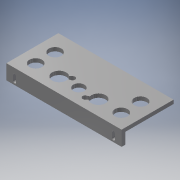
# Autodesk Inventor part: frontPanel
Saved by Autodesk Inventor 2017 (Build 210142000, 142)
## iProperties
Created: 2019-11-20
Part Number: frontPanel
Material: S235
Document SubType Name: Modeling
Designer: Casper
Density: 7.86 g/cm^3
Appearance: Steel
Author: Casper
Autodesk Inventor part; units mm, degrees
ref_plane "YZ Plane" through (0, 0, 0) normal (1, 0, 0) x (0, 1, 0)
ref_plane "XZ Plane" through (0, 0, 0) normal (0, 1, 0) x (-1, 0, 0)
ref_plane "XY Plane" through (0, 0, 0) normal (0, 0, 1) x (1, 0, 0)
sketch "Sketch1" plane through (0, 0, 0) normal (0, 0, 1) x (1, 0, 0)
  line L0 (-77.5, -35) -> (77.5, -35)
  line L1 (77.5, -35) -> (77.5, 35)
  line L2 (77.5, 35) -> (-77.5, 35)
  line L3 (-77.5, 35) -> (-77.5, -35)
  line L4 (-77.5, -35) -> (77.5, 35) construction
  line L5 (77.5, -35) -> (-77.5, 35) construction
  point P0 (0, 0)
  dimension "d23" = 155
  dimension "d24" = 70
  constraints: 12 end point, 2 midpoint, 2 parallel, 1 horizontal, 1 perpendicular
  measures "d23" distance of L0.start L0.end
  measures "d24" distance of L2.end L0.start
extrude "Extrusion2" add sketch "Sketch1" along normal blind 5
sketch "Sketch2" plane through (0, 0, 5) normal (0, 0, 1) x (1, 0, 0)
  line L0 (-77.5, -35) -> (77.5, -35) projected
  line L1 (77.5, -35) -> (77.5, 35) projected
  line L2 (77.5, 35) -> (-77.5, 35) projected
  line L3 (-77.5, 35) -> (-77.5, -35) projected
  line L4 (-77.5, -15) -> (77.5, -15) construction
  line L5 (77.5, -35) -> (77.5, 35) construction
  circle A0 centre (0, -15) radius 7.5
  circle A1 centre (26.5, -15) radius 9.5
  line L6 (0, 35) -> (0, -35) construction
  line L7 (-77.5, -35) -> (77.5, -35) construction
  circle A2 centre (-26.5, -15) radius 9.5
  circle A3 centre (15.5455, -22) radius 3.5
  circle A4 centre (-15.5455, -8) radius 3.5
  point P0 (0, 0)
  dimension "d27" = 20
  dimension "d28" = 15
  dimension "d29" = 19
  dimension "d30" = 26.5
  dimension "d31" = 7
  dimension "d32" = 7
  dimension "d33" = 7
  constraints: 5 centre point, 4 end point, 3 midpoint, 3 point on line, 2 tangent, 1 equal radius, 1 perpendicular, 1 symmetric about line, 1 other
  measures "d27" distance between parallel lines of L0 L4
  measures "d28" diameter of A0
  measures "d29" diameter of A1
  measures "d30" distance of A1.centre A0.centre
  measures "d31" diameter of A4
  measures "d32" vertical distance of A4.centre A2.centre
  measures "d33" vertical distance of A1.centre A3.centre
extrude "Extrusion3" cut sketch "Sketch2" against normal through all contours A0 | A1 | A3 | A2 | A4
sketch "Sketch3" plane through (0, 0, 5) normal (0, 0, 1) x (1, 0, 0)
  circle A0 centre (-26.5, -15) radius 9.5 projected
  circle A1 centre (-15.5455, -8) radius 3.5 projected
  circle A2 centre (26.5, -15) radius 9.5 projected
  circle A3 centre (15.5455, -22) radius 3.5 projected
  circle A4 centre (0, -15) radius 7.5 projected
  line L0 (-77.5, -35) -> (77.5, -35) projected
  line L1 (77.5, -35) -> (77.5, 35) projected
  line L2 (77.5, 35) -> (-77.5, 35) projected
  line L3 (-77.5, 35) -> (-77.5, -35) projected
  circle A5 centre (-26.5, -15) radius 9.5 projected
  line L4 (-20.5198, -7.6184) -> (-18.68, -6.4428)
  circle A6 centre (-15.5455, -8) radius 3.5 projected
  line L5 (-15.5455, -8) -> (-26.5, -15) construction
  line L6 (15.5455, -22) -> (26.5, -15) construction
  circle A7 centre (15.5455, -22) radius 3.5 projected
  line L7 (15.4493, -18.5013) -> (17.2891, -17.3257)
  line L8 (-17.2891, -12.6743) -> (-15.4493, -11.4987)
  line L9 (18.68, -23.5572) -> (20.5198, -22.3816)
  point P0 (0, 0)
  point P1 (-18.4948, -9.8846)
  point P2 (18.4948, -20.1154)
  dimension "d36" = 3
  dimension "d37" = 3
  dimension "d38" = 3
  dimension "d39" = 3
  constraints: 14 point on circle, 12 end point, 4 parallel
  measures "d36" distance between parallel lines of L4 L5
  measures "d37" distance between parallel lines of L7 L6
  measures "d38" distance between parallel lines of L8 L5
  measures "d39" distance between parallel lines of L9 L6
extrude "Extrusion4" cut sketch "Sketch3" against normal through all contours A0 A1 L8 | L4 A1 A0 | A2 A3 L7 | L9 A3 A2
sketch "Sketch4" plane through (0, 0, 5) normal (0, 0, 1) x (1, 0, 0)
  line L0 (-15.4493, -11.4987) -> (-17.2891, -12.6743) projected
  arc A0 (-20.5198, -7.6184) -> (-17.2891, -12.6743) centre (-26.5, -15) ccw projected
  line L1 (-20.5198, -7.6184) -> (-18.68, -6.4428) projected
  arc A1 (-15.4493, -11.4987) -> (-18.68, -6.4428) centre (-15.5455, -8) ccw projected
  line L2 (15.4493, -18.5013) -> (17.2891, -17.3257) projected
  arc A2 (20.5198, -22.3816) -> (17.2891, -17.3257) centre (26.5, -15) ccw projected
  line L3 (20.5198, -22.3816) -> (18.68, -23.5572) projected
  arc A3 (15.4493, -18.5013) -> (18.68, -23.5572) centre (15.5455, -22) ccw projected
  circle A4 centre (0, -15) radius 7.5 projected
  line L4 (-77.5, -35) -> (77.5, -35) projected
  line L5 (77.5, -35) -> (77.5, 35) projected
  line L6 (77.5, 35) -> (-77.5, 35) projected
  line L7 (-77.5, 35) -> (-77.5, -35) projected
  line L8 (-77.5, -25) -> (77.5, -25) construction
  line L9 (-67.5, -25) -> (-47.5, -25) construction
  line L10 (-47.5, -25) -> (-47.5, 20) construction
  line L11 (-47.5, 20) -> (-67.5, 20) construction
  line L12 (-67.5, 20) -> (-67.5, -25) construction
  line L13 (77.5, 35) -> (-77.5, 35) construction
  line L14 (0, 35) -> (0, -35) construction
  circle A5 centre (-57.5, 10.5) radius 8.5
  circle A6 centre (-57.5, -15.5) radius 8.5
  line L15 (-67.5, -2.5) -> (-47.5, -2.5) construction
  line L16 (-57.5, -2.5) -> (-57.5, 10.5) construction
  line L17 (-57.5, -2.5) -> (-57.5, -15.5) construction
  circle A7 centre (57.5, 10.5) radius 8.5
  circle A8 centre (57.5, -15.5) radius 8.5
  point P0 (0, 0)
  dimension "d42" = 10
  dimension "d43" = 10
  dimension "d44" = 20
  dimension "d45" = 45
  dimension "d46" = 17
  dimension "d48" = 26
  constraints: 18 end point, 5 midpoint, 4 centre point, 3 point on line, 2 parallel, 2 perpendicular, 2 symmetric about line, 2 vertical, 1 collinear, 1 equal radius, 1 horizontal, 2 other
  measures "d42" distance between parallel lines of L4 L8
  measures "d43" distance between parallel lines of L7 L12
  measures "d44" distance of L10.end L11.end
  measures "d45" distance of L9.end L10.end
  measures "d46" diameter of A5
  measures "d48" distance of L17.end L16.end
extrude "Extrusion5" cut sketch "Sketch4" against normal through all contours A5 | A6 | A7 | A8
sketch "Sketch5" plane through (0, 0, 0) normal (0, 0, -1) x (-1, 0, 0)
  circle A0 centre (-57.5, 10.5) radius 8.5 projected
  circle A1 centre (57.5, 10.5) radius 8.5 projected
  circle A2 centre (57.5, -15.5) radius 8.5 projected
  circle A3 centre (-57.5, -15.5) radius 8.5 projected
  line L0 (17.2891, -12.6743) -> (15.4493, -11.4987) projected
  arc A4 (18.68, -6.4428) -> (15.4493, -11.4987) centre (15.5455, -8) ccw projected
  line L1 (18.68, -6.4428) -> (20.5198, -7.6184) projected
  arc A5 (17.2891, -12.6743) -> (20.5198, -7.6184) centre (26.5, -15) ccw projected
  line L2 (-17.2891, -17.3257) -> (-15.4493, -18.5013) projected
  arc A6 (-18.68, -23.5572) -> (-15.4493, -18.5013) centre (-15.5455, -22) ccw projected
  line L3 (-18.68, -23.5572) -> (-20.5198, -22.3816) projected
  arc A7 (-17.2891, -17.3257) -> (-20.5198, -22.3816) centre (-26.5, -15) ccw projected
  circle A8 centre (0, -15) radius 7.5 projected
  line L4 (77.5, -35) -> (-77.5, -35) projected
  line L5 (77.5, 35) -> (77.5, -35) projected
  line L6 (-77.5, 35) -> (77.5, 35) projected
  line L7 (-77.5, -35) -> (-77.5, 35) projected
  line L8 (-77.5, -30) -> (77.5, -30)
  line L9 (77.5, 35) -> (77.5, -35) construction
  line L10 (-77.5, -30) -> (77.5, -30)
  line L11 (77.5, -30) -> (77.5, -35)
  line L12 (77.5, -35) -> (-77.5, -35)
  line L13 (-77.5, -35) -> (-77.5, -30)
  point P0 (0, 0)
  dimension "d51" = 5
  constraints: 10 end point, 2 parallel, 2 perpendicular, 2 point on line, 1 horizontal
  measures "d51" distance between parallel lines of L4 L8
extrude "Extrusion6" add sketch "Sketch5" along normal blind 15 contours L4 L7 L8 L5
sketch "Sketch6" plane through (-77.5, -30, 0) normal (0, 1, 0) x (1, 0, 0)
  line L0 (155, 0) -> (0, 0) projected
  line L1 (155, 0) -> (155, 15) projected
  line L2 (0, 15) -> (155, 15) projected
  line L3 (0, 0) -> (0, 15) projected
  line L4 (146, 4) -> (142, 4)
  line L5 (142, 4) -> (142, 11)
  line L6 (142, 11) -> (146, 11)
  line L7 (146, 11) -> (146, 4)
  arc A0 (142, 4) -> (146, 4) centre (144, 4) ccw
  arc A1 (146, 11) -> (142, 11) centre (144, 11) ccw
  line L8 (155, 15) -> (0, 15) construction
  line L9 (77.5, 15) -> (77.5, 0) construction
  line L10 (9, 4) -> (13, 4)
  line L11 (13, 4) -> (13, 11)
  line L12 (13, 11) -> (9, 11)
  line L13 (9, 11) -> (9, 4)
  arc A2 (9, 4) -> (13, 4) centre (11, 4) ccw
  arc A3 (13, 11) -> (9, 11) centre (11, 11) ccw
  point P0 (146, 7.5)
  point P1 (155, 7.5)
  point P2 (9, 7.5)
  dimension "d54" = 4
  dimension "d55" = 7
  dimension "d56" = 9
  constraints: 18 end point, 8 point on circle, 7 symmetric about line, 5 midpoint, 4 centre point, 2 parallel, 1 horizontal, 1 horizontal alignment, 1 perpendicular, 1 vertical, 2 other
  measures "d54" distance between parallel lines of L7 L5
  measures "d55" distance of L4.end L5.end
  measures "d56" distance between parallel lines of L1 L7
extrude "Extrusion7" cut sketch "Sketch6" against normal through all contours A0 L4 | L4 L5 L6 L7 | L6 A1 | L13 L12 L11 L10 | L10 A2 | A3 L12
body "Solid2"
